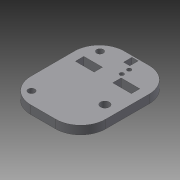
# Autodesk Inventor part: Carriage_Frame
Saved by Autodesk Inventor 2014 (Build 180170000, 170)
## iProperties
Created: 2014-08-27
Part Number: Carriage_Frame
Material: Generic
Document SubType Name: Modeling
Designer: ThatOtherGuy
Density: 1 g/cm^3
Appearance: Default
Author: ThatOtherGuy
Autodesk Inventor part; units mm, degrees
ref_plane "YZ Plane" through (0, 0, 0) normal (1, 0, 0) x (0, 1, 0)
ref_plane "XZ Plane" through (0, 0, 0) normal (0, 1, 0) x (-1, 0, 0)
ref_plane "XY Plane" through (0, 0, 0) normal (0, 0, 1) x (1, 0, 0)
sketch "Sketch1" plane through (0, 0, 0) normal (0, 0, 1) x (1, 0, 0)
  circle A0 centre (10.5, 65) radius 2.65
  circle A1 centre (10.5, 10) radius 2.65
  circle A2 centre (49.5, 30) radius 3.5
  line L0 (60, 75) -> (60, 0)
  line L1 (60, 0) -> (0, 0)
  line L2 (0, 0) -> (0, 75)
  line L3 (0, 75) -> (60, 75)
  point P0 (30, 75)
  dimension "d0" = 39
  dimension "d1" = 5.3
  dimension "d2" = 55
  dimension "d3" = 10
  dimension "d5" = 10.5
  dimension "d16" = 10.5
  dimension "d19" = 20
  dimension "d22" = 7
  dimension "d55" = 75
  dimension "d64" = 60
  constraints: 10 end point, 3 centre point, 2 perpendicular, 1 coincident, 1 equal radius, 1 horizontal, 1 midpoint, 1 parallel, 1 vertical alignment
  measures "d0" horizontal distance of A0.centre A2.centre
  measures "d1" diameter of A0
  measures "d2" distance of A0.centre A1.centre
  measures "d3" distance from line of L1 A1.centre
  measures "d5" distance from line of L0 A2.centre
  measures "d16" distance from line of L2 A1.centre
  measures "d19" vertical distance of A2.centre A1.centre
  measures "d22" diameter of A2
  measures "d55" distance between parallel lines of L1 L3
  measures "d64" distance of L2.end L0.start
extrude "Extrusion1" add sketch "Sketch1" along normal blind 6.731
sketch "Sketch3" plane through (0, 0, 6.731) normal (0, 0, 1) x (1, 0, 0)
  line L0 (60, 0) -> (60, 75) projected
  line L1 (60, 75) -> (0, 75) projected
  line L2 (0, 75) -> (0, 0) projected
  line L3 (7.5, 55) -> (22.5, 55)
  line L4 (22.5, 55) -> (22.5, 48.269)
  line L5 (22.5, 48.269) -> (7.5, 48.269)
  line L6 (7.5, 48.269) -> (7.5, 55)
  line L7 (37.5, 55) -> (52.5, 55)
  line L8 (52.5, 55) -> (52.5, 48.269)
  line L9 (52.5, 48.269) -> (37.5, 48.269)
  line L10 (37.5, 48.269) -> (37.5, 55)
  line L11 (27.5, 73.731) -> (32.5, 73.731)
  line L12 (32.5, 73.731) -> (32.5, 67)
  line L13 (32.5, 67) -> (27.5, 67)
  line L14 (27.5, 67) -> (27.5, 73.731)
  circle A0 centre (35, 64) radius 1.588
  circle A1 centre (35, 58) radius 1.588
  line L15 (37.5, 55) -> (30, 55) construction
  line L16 (30, 55) -> (22.5, 55) construction
  point P0 (30, 67)
  dimension "d70" = 15
  dimension "d71" = 6.731
  dimension "d73" = 15
  dimension "d74" = 7.5
  dimension "d75" = 7.5
  dimension "d78" = 20
  dimension "d81" = 12
  dimension "d84" = 3.176
  dimension "d91" = 3
  dimension "d92" = 6
  dimension "d93" = 3
  dimension "d94" = 5
  dimension "d95" = 5
  constraints: 28 end point, 6 parallel, 3 collinear, 3 equal length, 3 horizontal, 3 perpendicular, 2 centre point, 2 vertical alignment, 1 equal radius, 1 midpoint
  measures "d70" distance of L3.start L3.end
  measures "d71" distance of L5.end L3.start
  measures "d73" distance between parallel lines of L10 L4
  measures "d74" distance between parallel lines of L2 L6
  measures "d75" distance between parallel lines of L0 L8
  measures "d78" distance between parallel lines of L1 L3
  measures "d81" distance between parallel lines of L7 L13
  measures "d84" diameter of A1
  measures "d91" distance from line of L15 A1.centre
  measures "d92" distance of A0.centre A1.centre
  measures "d93" distance from line of L13 A0.centre
  measures "d94" distance of L11.start L11.end
  measures "d95" horizontal distance of L15.end A1.centre
extrude "Extrusion3" cut sketch "Sketch3" against normal up to next
fillet "Fillet2" radius 20 2 edges at (60, 0, 3.3655) (0, 0, 3.3655)
fillet "Fillet2" radius 20 2 edges at (0, 75, 3.3655) (60, 75, 3.3655)
equation "\"d16\" = d5"
equation "\"d20\" = THICKB"
equation "\"THICKA\" = 3.175"
equation "\"THICKB\" = 6.731"
equation "\"THICKC\" = 12.7"
equation "\"BALLDIA\" = 12"
equation "\"MAGDIA\" = 9.5"
equation "\"THICKPLY\" = 5"
body "Solid1"
